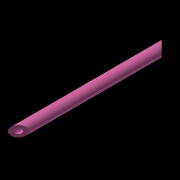
# Autodesk Inventor part: Long Pool Noodle
Saved by Autodesk Inventor 2014 SP1 (Build 180222100, 222)
## iProperties
Created: 2013-11-30
Part Number: Long Pool Noodle
Material: Generic
Document SubType Name: Modeling
Designer: Rauhul Varma
Mass: 2133.01 g
Surface Area: 2514.4 cm^2
Volume: 2133.01 cm^3
Density: 1 g/cm^3
Appearance: Pink
Author: Rauhul Varma
Autodesk Inventor part; units mm, degrees
ref_plane "YZ Plane" through (0, 0, 0) normal (1, 0, 0) x (0, 1, 0)
ref_plane "XZ Plane" through (0, 0, 0) normal (0, 1, 0) x (-1, 0, 0)
ref_plane "XY Plane" through (0, 0, 0) normal (0, 0, 1) x (1, 0, 0)
sketch "Sketch1" plane through (0, 0, 0) normal (0, 0, 1) x (1, 0, 0)
  circle A0 centre (0, 0) radius 31.75
  circle A1 centre (0, 0) radius 14.2875
  dimension "d0" = 63.5
  dimension "d1" = 28.575
  constraints: 2 centre point, 2 coincident
  measures "d0" diameter of A0
  measures "d1" diameter of A1
extrude "Extrusion1" add sketch "Sketch1" along normal blind 908.05
sketch "Sketch3" plane through (0, 0, 0) normal (0, 1, 0) x (-1, 0, 0)
  line L0 (-31.75, 0) -> (-31.75, 908.05) projected
  line L1 (-31.75, 0) -> (31.75, 0) projected
  line L2 (31.75, 0) -> (31.75, 908.05) projected
  line L3 (31.75, 908.05) -> (-31.75, 908.05) projected
  line L4 (31.75, 908.05) -> (-31.75, 844.55)
  line L5 (31.75, 908.05) -> (121.5526, 908.05) construction
  line L6 (31.75, 0) -> (-31.75, 63.5)
  line L7 (31.75, 0) -> (121.5526, 0) construction
  point P0 (0, 0)
  dimension "d6" = 135
  dimension "d7" = 135
  constraints: 8 end point, 2 equal length, 2 horizontal, 2 point on line
  measures "d6" angle of L4 L5
  measures "d7" angle of L7 L6
extrude "Extrusion2" cut sketch "Sketch3" along normal through all both and the other way through all contours L0 L6 L1 | L0 L3 L4
body "Solid1"
